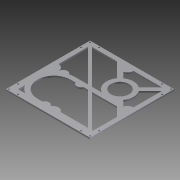
# Autodesk Inventor part: upper gearbox bottom plate
Saved by Autodesk Inventor 2012 (Build 160160000, 160)
## iProperties
Created: 2012-07-07
Part Number: upper gearbox bottom plate
Material: Default
Document SubType Name: Modeling
Designer: Bryce
Density: 1 g/cm^3
Author: Bryce
Autodesk Inventor part; units mm, degrees
ref_plane "YZ Plane" through (0, 0, 0) normal (1, 0, 0) x (0, 1, 0)
ref_plane "XZ Plane" through (0, 0, 0) normal (0, 1, 0) x (-1, 0, 0)
ref_plane "XY Plane" through (0, 0, 0) normal (0, 0, 1) x (1, 0, 0)
sketch "Sketch1" plane through (0, 0, 0) normal (0, 0, 1) x (1, 0, 0)
  line L0 (-114.3, 114.3) -> (63.5, 114.3)
  line L1 (63.5, 114.3) -> (63.5, -63.5)
  line L2 (63.5, -63.5) -> (-114.3, -63.5)
  line L3 (-114.3, -63.5) -> (-114.3, 114.3)
  circle A0 centre (6.35, -6.35) radius 19.05
  circle A1 centre (41.275, 111.125) radius 1.5875
  circle A2 centre (60.325, -41.275) radius 1.5875
  circle A3 centre (-92.075, -60.325) radius 1.5875
  circle A4 centre (-111.125, 92.075) radius 1.5875
  circle A5 centre (-111.125, 111.125) radius 1.5875
  circle A6 centre (-92.075, 111.125) radius 1.5875
  circle A7 centre (60.325, 92.075) radius 1.5875
  circle A8 centre (60.325, -60.325) radius 1.5875
  circle A9 centre (41.275, -60.325) radius 1.5875
  circle A10 centre (-111.125, -60.325) radius 1.5875
  circle A11 centre (-111.125, -41.275) radius 1.5875
  circle A12 centre (60.325, 111.125) radius 1.5875
  arc A13 (-92.7105, 44.3557) -> (-34.2895, 44.3557) centre (-63.5, 63.5) ccw construction
  line L4 (-98.425, 63.5) -> (-28.575, 63.5)
  line L5 (-28.575, 63.5) -> (-28.575, 52.7537)
  line L6 (-98.425, -53.975) -> (-98.425, -52.1151)
  line L7 (53.975, -53.975) -> (6.35, -6.35) construction
  line L8 (22.9054, -29.6406) -> (47.2398, -53.975)
  line L9 (47.2398, -53.975) -> (-12.7, -53.975)
  line L10 (6.35, -6.35) -> (40.026, 27.326) construction
  line L11 (29.6406, 10.2054) -> (41.6746, 22.2394)
  arc A14 (29.6406, -22.9054) -> (29.6406, 10.2054) centre (6.35, -6.35) ccw
  line L12 (29.6406, -22.9054) -> (53.975, -47.2398)
  line L13 (-19.05, 27.2599) -> (-19.05, 6.7409)
  arc A15 (22.9054, 16.9406) -> (-19.05, 6.7409) centre (6.35, -6.35) ccw
  line L14 (-101.6, 101.6) -> (-86.3953, 101.6)
  line L15 (-101.6, 86.3953) -> (-101.6, 101.6)
  arc A16 (-86.3953, 101.6) -> (-101.6, 86.3953) centre (-63.5, 63.5) ccw
  arc A17 (-19.05, 63.5) -> (-20.4156, 74.4333) centre (-63.5, 63.5) ccw
  line L16 (-19.05, 36.2401) -> (-19.05, 63.5)
  arc A18 (-20.4156, 74.4333) -> (-25.4, 92.075) centre (-25.4, 82.55) ccw
  arc A19 (-28.575, 52.7537) -> (-28.575, 36.1463) centre (-25.4, 44.45) ccw
  line L17 (-28.575, 36.1463) -> (-28.575, 26.7151)
  line L18 (-98.425, 52.7537) -> (-98.425, 63.5)
  arc A20 (-30.6583, 51.6182) -> (-98.425, 63.5) centre (-63.5, 63.5) ccw
  line L19 (6.35, -6.35) -> (-25.0809, -37.7809) construction
  line L20 (-10.2054, -29.6406) -> (-22.2394, -41.6746)
  arc A21 (-10.2054, -29.6406) -> (22.9054, -29.6406) centre (6.35, -6.35) ccw
  line L21 (-28.575, -34.5398) -> (-48.0102, -53.975)
  line L22 (-48.0102, -53.975) -> (-98.425, -53.975)
  line L23 (-25.0809, -37.7809) -> (-43.0414, -55.7414) construction
  line L24 (40.026, 27.326) -> (57.9865, 45.2865)
  line L25 (57.9865, 45.2865) -> (53.975, 41.275)
  arc A22 (-12.7, -53.975) -> (-22.2394, -41.6746) centre (-25.4, -53.975) ccw
  arc A23 (41.6746, 22.2394) -> (53.975, 12.7) centre (53.975, 25.4) ccw
  line L26 (53.975, 12.7) -> (53.975, -47.2398)
  arc A24 (-98.425, 14.4015) -> (-98.171, 36.2479) centre (-104.775, 25.4) ccw
  arc A25 (-98.171, 36.2479) -> (-98.425, 52.7537) centre (-101.6, 44.45) ccw
  line L27 (53.975, 48.0102) -> (53.975, 100.2849)
  line L28 (-12.7, 104.775) -> (49.4849, 104.775)
  arc A26 (-98.425, 63.5) -> (-96.3417, 51.6182) centre (-63.5, 63.5) ccw construction
  arc A27 (-25.4, 92.075) -> (-12.7, 104.775) centre (-25.4, 104.775) ccw
  line L29 (-114.3, -63.5) -> (63.5, 114.3) construction
  line L30 (-98.425, -43.1349) -> (-28.575, 26.7151)
  line L31 (-98.425, -52.1151) -> (-28.575, 17.7349)
  line L32 (22.9054, 16.9406) -> (53.975, 48.0102)
  line L33 (-19.05, 36.2401) -> (49.4849, 104.775)
  line L34 (-19.05, 27.2599) -> (53.975, 100.2849)
  line L35 (-28.575, 17.7349) -> (-28.575, -34.5398)
  line L36 (-28.575, 26.7151) -> (-28.575, 17.7349) construction
  line L37 (49.4849, 104.775) -> (53.975, 104.775) construction
  line L38 (53.975, 100.2849) -> (53.975, 104.775) construction
  line L39 (-98.425, -52.1151) -> (-98.425, -43.1349) construction
  line L40 (-98.425, -43.1349) -> (-98.425, 14.4015)
  line L41 (-25.4, -53.975) -> (-104.775, 25.4) construction
  point P0 (0, 0)
  point P1 (-101.6, 82.55)
  dimension "d0" = 114.3
  dimension "d1" = 177.8
  dimension "d2" = 177.8
  dimension "d3" = 114.3
  dimension "d4" = 38.1
  dimension "d5" = 57.15
  dimension "d6" = 57.15
  dimension "d10" = 3.175
  dimension "d11" = 3.175
  dimension "d12" = 3.175
  dimension "d15" = 3.175
  dimension "d16" = 22.225
  dimension "d17" = 22.225
  dimension "d18" = 3.175
  dimension "d19" = 3.175
  dimension "d20" = 22.225
  dimension "d23" = 3.175
  dimension "d24" = 3.175
  dimension "d25" = 22.225
  dimension "d26" = 3.175
  dimension "d27" = 3.175
  dimension "d28" = 3.175
  dimension "d29" = 3.175
  dimension "d30" = 22.225
  dimension "d34" = 3.175
  dimension "d35" = 3.175
  dimension "d36" = 3.175
  dimension "d37" = 3.175
  dimension "d38" = 22.225
  dimension "d39" = 3.175
  dimension "d40" = 3.175
  dimension "d41" = 3.175
  dimension "d42" = 3.175
  dimension "d43" = 3.175
  dimension "d44" = 3.175
  dimension "d45" = 3.175
  dimension "d46" = 22.225
  dimension "d47" = 3.175
  dimension "d48" = 3.175
  dimension "d49" = 3.175
  dimension "d50" = 3.175
  dimension "d51" = 22.225
  dimension "d52" = 3.175
  dimension "d55" = 69.85
  dimension "d56" = 50.8
  dimension "d57" = 50.8
  dimension "d93" = 69.85
  dimension "d94" = 15.875
  dimension "d97" = 38.1
  dimension "d98" = 38.1
  dimension "d99" = 38.1
  dimension "d100" = 38.1
  dimension "d101" = 19.05
  dimension "d102" = 19.05
  dimension "d103" = 19.05
  dimension "d104" = 19.05
  dimension "d212" = 9.525
  dimension "d216" = 4.7625
  dimension "d218" = 45
  dimension "d222" = 6.7352
  dimension "d226" = 28.575
  dimension "d227" = 4.7625
  dimension "d228" = 4.7625
  dimension "d232" = 9.525
  constraints: 85 end point, 35 point on circle, 32 parallel, 28 centre point, 12 coincident, 12 perpendicular, 7 point on line, 3 horizontal, 2 vertical alignment, 1 collinear, 1 vertical
  measures "d0" distance from line of L0 point (0, 0)
  measures "d1" distance of L0.end L1.end
  measures "d2" distance of L0.start L0.end
  measures "d3" distance from line of L3 point (0, 0)
  measures "d4" diameter of A0
  measures "d5" distance from line of L1 L7.end
  measures "d6" distance from line of L2 L7.end
  measures "d10" diameter of A1
  measures "d11" diameter of A2
  measures "d12" diameter of A3
  measures "d15" distance from line of L0 A1.centre
  measures "d16" distance from line of L1 A1.centre
  measures "d17" distance from line of L2 A2.centre
  measures "d18" distance from line of L1 A2.centre
  measures "d19" distance from line of L2 A3.centre
  measures "d20" distance from line of L3 A3.centre
  measures "d23" diameter of A4
  measures "d24" distance from line of L3 A4.centre
  measures "d25" distance from line of L0 A4.centre
  measures "d26" diameter of A5
  measures "d27" distance from line of L0 A5.centre
  measures "d28" distance from line of L3 A5.centre
  measures "d29" distance from line of L0 A6.centre
  measures "d30" distance from line of L3 A6.centre
  measures "d34" diameter of A12
  measures "d35" distance from line of L0 A12.centre
  measures "d36" distance from line of L1 A12.centre
  measures "d37" distance from line of L1 A7.centre
  measures "d38" distance from line of L0 A7.centre
  measures "d39" diameter of A7
  measures "d40" diameter of A6
  measures "d41" diameter of A8
  measures "d42" distance from line of L1 A8.centre
  measures "d43" distance from line of L2 A8.centre
  measures "d44" diameter of A9
  measures "d45" distance from line of L2 A9.centre
  measures "d46" distance from line of L1 A9.centre
  measures "d47" diameter of A10
  measures "d48" distance from line of L2 A10.centre
  measures "d49" distance from line of L3 A10.centre
  measures "d50" diameter of A11
  measures "d51" distance from line of L2 A11.centre
  measures "d52" distance from line of L3 A11.centre
  measures "d55" diameter of A13
  measures "d56" distance from line of L0 A13.centre
  measures "d57" distance from line of L3 A13.centre
  measures "d93" distance of L4.start L4.end
  measures "d94" distance between parallel lines of L3 L6
  measures "d97" horizontal distance of A13.centre point (-101.6, 82.55)
  measures "d98" horizontal distance of A13.centre point (-101.6, 44.45)
  measures "d99" horizontal distance of point (-25.4, 82.55) A13.centre
  measures "d100" horizontal distance of point (-25.4, 44.45) A13.centre
  measures "d101" vertical distance of point (-101.6, 82.55) A13.centre
  measures "d102" vertical distance of A13.centre point (-101.6, 44.45)
  measures "d103" vertical distance of point (-25.4, 44.45) A13.centre
  measures "d104" vertical distance of point (-25.4, 82.55) A13.centre
  measures "d212" distance from line of L1 L7.start
  measures "d216" distance between parallel lines of L7 L8
  measures "d218" angle of L9 L8
  measures "d222" distance of L7.start L8.end
  measures "d226" radius of A14
  measures "d227" distance between parallel lines of L12 L7
  measures "d228" distance between parallel lines of L10 L11
  measures "d232" distance between parallel lines of L13 L5
extrude "Extrusion12" [suppressed]
extrude "Extrusion13" [suppressed]
hole "Hole9" [suppressed]
extrude "Extrusion14" [suppressed]
fillet "Fillet2" [suppressed]
fillet "Fillet3" [suppressed]
extrude "Extrusion15" [suppressed]
fillet "Fillet4" [suppressed]
hole "Hole10" [suppressed]
hole "Hole11" [suppressed]
hole "Hole12" [suppressed]
chamfer "Chamfer1" [suppressed]
chamfer "Chamfer2" [suppressed]
extrude "Extrusion16" [suppressed]
fillet "Fillet6" [suppressed]
extrude "Extrusion17" add sketch "Sketch1" along normal blind 3.175
body "Solid7"
